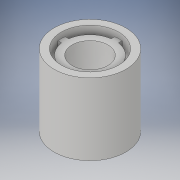
# Autodesk Inventor part: Connector_box_inner_part
Saved by Autodesk Inventor 2019.3 (Build 233278000, 278)
## iProperties
Created: 2019-02-06
Part Number: Connector_box_inner_part
Material: Generic
Document SubType Name: Modeling
Designer: Varga Daniel
Density: 1 g/cm^3
Appearance: Default
Author: Varga Daniel
Autodesk Inventor part; units mm, degrees
ref_plane "YZ Plane" through (0, 0, 0) normal (1, 0, 0) x (0, 1, 0)
ref_plane "XZ Plane" through (0, 0, 0) normal (0, 1, 0) x (-1, 0, 0)
ref_plane "XY Plane" through (0, 0, 0) normal (0, 0, 1) x (1, 0, 0)
derived "beam_single_end_part.ipt"
sketch "Sketch3" plane through (0, 0, 0) normal (0, 1, 0) x (-1, 0, 0)
  circle A0 centre (5, 5) radius 2.5 construction
  circle A1 centre (5, 5) radius 3.5 construction
  arc A2 (2.5, 5) -> (5, 7.5) centre (5, 5) ccw
  arc A3 (4.5, 1.5359) -> (5.5, 1.5359) centre (5, 5) ccw
  line L0 (0.3508, 5) -> (13.598, 5) construction
  line L1 (5, 13.9543) -> (5, -1.7484) construction
  line L2 (5, 10) -> (0, 10)
  line L3 (0, 10) -> (0, 9)
  line L4 (0, 9) -> (0, 9)
  line L5 (0, 1) -> (0, 0)
  line L6 (0, 0) -> (5, 0)
  line L7 (0, 0) -> (0, 1)
  line L8 (1.5359, 5.5) -> (0, 5.5)
  line L9 (0, 5.5) -> (0, 4.5)
  line L10 (0, 4.5) -> (1.5359, 4.5)
  line L11 (0, 9) -> (4.5, 9)
  line L12 (0, 9) -> (0, 10)
  line L13 (5, 9) -> (5, 9)
  line L14 (5, 1) -> (4.5, 1)
  arc A4 (5, 1) -> (5.5, 1.0314) centre (5, 5) ccw
  line L15 (4.5, 9) -> (4.5, 8.4641)
  line L16 (5.5, 8.9686) -> (5.5, 8.4641)
  line L17 (5.5, 1.0314) -> (5.5, 1.5359)
  line L18 (4.5, 1.5359) -> (4.5, 1)
  line L19 (8.4641, 5.5) -> (8.9686, 5.5)
  line L20 (8.4641, 4.5) -> (8.9686, 4.5)
  line L21 (0, 1) -> (0, 4.5)
  line L22 (0, 4.5) -> (0, 5.5)
  line L23 (0, 5.5) -> (0, 9)
  line L24 (4.5, 9) -> (5, 9)
  arc A5 (8.9686, 5.5) -> (5.5, 8.9686) centre (5, 5) ccw
  arc A6 (8.9686, 4.5) -> (8.9686, 5.5) centre (5, 5) ccw
  arc A7 (1.5359, 4.5) -> (4.5, 1.5359) centre (5, 5) ccw
  arc A8 (1.5359, 5.5) -> (1.5359, 4.5) centre (5, 5) ccw
  line L25 (4.5, 1) -> (0, 1)
  line L26 (0, 9) -> (4.5, 9)
  line L27 (4.5, 9) -> (5, 9)
  circle A9 centre (5, 5) radius 2.5 construction
  arc A10 (10, 5) -> (5, 10) centre (5, 5) ccw
  arc A11 (5, 0) -> (10, 5) centre (5, 5) ccw
  arc A12 (5.5, 8.9686) -> (5, 9) centre (5, 5) ccw
  arc A13 (8.4641, 5.5) -> (5.5, 8.4641) centre (5, 5) ccw
  arc A14 (5.5, 8.4641) -> (4.5, 8.4641) centre (5, 5) ccw
  arc A15 (5.5, 1.0314) -> (8.9686, 4.5) centre (5, 5) ccw
  arc A16 (8.4641, 4.5) -> (8.4641, 5.5) centre (5, 5) ccw
  arc A17 (4.5, 8.4641) -> (1.5359, 5.5) centre (5, 5) ccw
  arc A18 (5.5, 1.5359) -> (8.4641, 4.5) centre (5, 5) ccw
  arc A19 (5, 7.5) -> (2.5, 5) centre (5, 5) ccw
  point P0 (0, 0)
sketch "Sketch2" plane through (0, 0, 0) normal (0, 1, 0) x (-1, 0, 0)
  arc A0 (10, 5) -> (5, 10) centre (5, 5) ccw projected
  arc A1 (5, 0) -> (10, 5) centre (5, 5) ccw projected
  arc A2 (5.5, 1.0314) -> (8.9686, 4.5) centre (5, 5) ccw projected
  arc A3 (5, 1) -> (5.5, 1.0314) centre (5, 5) ccw projected
  line L0 (5.5, 1.0314) -> (5.5, 1.5359) projected
  arc A4 (4.5, 1.5359) -> (5.5, 1.5359) centre (5, 5) ccw projected
  circle A5 centre (5, 5) radius 3.5 projected
  circle A6 centre (5, 5) radius 2.5 projected
  line L1 (8.4641, 4.5) -> (8.9686, 4.5) projected
  line L2 (8.4641, 5.5) -> (8.9686, 5.5) projected
  arc A7 (8.9686, 5.5) -> (5.5, 8.9686) centre (5, 5) ccw projected
  arc A8 (5.5, 8.9686) -> (5, 9) centre (5, 5) ccw projected
  line L3 (5.5, 8.9686) -> (5.5, 8.4641) projected
  arc A9 (5.5, 8.4641) -> (4.5, 8.4641) centre (5, 5) ccw projected
  line L4 (5, 13.9543) -> (5, -1.7484) construction
  line L5 (0.3508, 5) -> (13.598, 5) construction
  arc A10 (5, 7.5) -> (2.5, 5) centre (5, 5) ccw projected
  arc A11 (4.5, 8.4641) -> (1.5359, 5.5) centre (5, 5) ccw projected
  arc A12 (1.5359, 5.5) -> (1.5359, 4.5) centre (5, 5) ccw projected
  arc A13 (8.9686, 4.5) -> (8.9686, 5.5) centre (5, 5) ccw projected
  arc A14 (8.4641, 4.5) -> (8.4641, 5.5) centre (5, 5) ccw projected
  arc A15 (5, 10) -> (0, 5) centre (5, 5) ccw
  arc A16 (0, 5) -> (5, 0) centre (5, 5) ccw
  arc A17 (1.0314, 4.5) -> (4.5, 1.0314) centre (5, 5) ccw
  arc A18 (4.5, 1.0314) -> (5, 1) centre (5, 5) ccw
  line L6 (4.5, 1.0314) -> (4.5, 1.5359)
  line L7 (1.5359, 4.5) -> (1.0314, 4.5)
  line L8 (1.5359, 5.5) -> (1.0314, 5.5)
  arc A19 (4.5, 8.9686) -> (1.0314, 5.5) centre (5, 5) ccw
  arc A20 (5, 9) -> (4.5, 8.9686) centre (5, 5) ccw
  line L9 (4.5, 8.9686) -> (4.5, 8.4641)
  arc A21 (1.0314, 5.5) -> (1.0314, 4.5) centre (5, 5) ccw
  arc A22 (1.5359, 5.5) -> (1.5359, 4.5) centre (5, 5) ccw
  point P0 (0, 0)
  constraints: 16 point on circle, 8 centre point, 8 end point, 5 symmetric about line, 9 other
extrude "Extrusion1" add sketch "Sketch2" along normal mid plane 8.4 contours A3 A18 L6 A4 L0 | L1 A5 L2 A13 | A4 A5 | L3 A5 L9 A20 A8 | A21 L8 A5 L7
extrude "Extrusion3" add sketch "Sketch2" along normal mid plane 10 contours A1 A16 A15 A0
extrude "Extrusion4" add sketch "Sketch2" along normal mid plane 1 contours L0 A5 L1 A2 | A3 A18 L6 A4 L0 | L1 A5 L2 A13 | A4 A5 | L2 A5 L3 A7 | A17 L7 A5 L6 | L3 A5 L9 A20 A8 | A21 L8 A5 L7 | A19 L9 A5 L8
equation "\"d1\" = Hole_height"
equation "\"d5\" = Overall_height"
equation "\"d7\" = Inner_thickness"
equation "\"Hole_height\" = 8.4"
equation "\"Overall_height\" = 10"
equation "\"Inner_thickness\" = 1"
body "Solid1"
